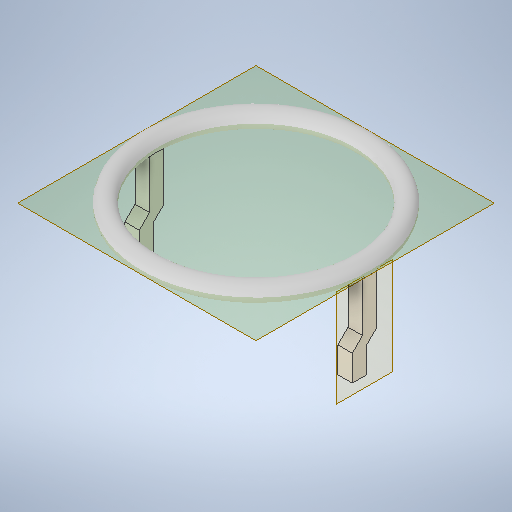
# Autodesk Inventor part: basket holder
Saved by Autodesk Inventor 2025.4 (Build 294407000, 407)
## iProperties
Created: 2026-03-21
Part Number: basket holder
Material: Generic
Document SubType Name: Modeling
Designer: Amir
Density: 1 g/cm^3
Appearance: Default
Author: Amir
Autodesk Inventor part; units mm, degrees
ref_plane "XZ Plane" through (0, 0, 0) normal (0, 1, 0) x (-1, 0, 0)
ref_plane "XY Plane" through (0, 0, 0) normal (0, 0, 1) x (1, 0, 0)
sketch "Sketch1" plane through (0, 0, 0) normal (0, 0, 1) x (1, 0, 0)
  circle A0 centre (0, 29.5) radius 2.5
  line L0 (-6.3664, 0) -> (5.4497, 0)
  point P0 (0, 0)
  dimension "d2" = 5
  dimension "d11" = 29.5
  constraints: 2 end point, 1 centre point, 1 horizontal
  measures "d2" diameter of A0
  measures "d11" distance from line of A0.centre L0
revolve "Revolution1" add sketch "Sketch1" angle 360 about axis through (-6.3664, 0, 0) along (1, 0, 0)
ref_plane "Work Plane1" through (0, 0, 0) normal (1, 0, 0) x (0, 1, 0)
sketch "Sketch2" plane through (0, 0, 0) normal (1, 0, 0) x (0, 1, 0)
  line L0 (2, -27.5) -> (-2, -27.5)
  line L1 (-2, -27.5) -> (-2, -31.5)
  line L2 (-2, -31.5) -> (2, -31.5)
  line L3 (2, -31.5) -> (2, -27.5)
  line L4 (2, -27.5) -> (-2, -31.5) construction
  line L5 (-2, -27.5) -> (2, -31.5) construction
  line L6 (2, 31.5) -> (-2, 31.5)
  line L7 (-2, 31.5) -> (-2, 27.5)
  line L8 (-2, 27.5) -> (2, 27.5)
  line L9 (2, 27.5) -> (2, 31.5)
  line L10 (2, 31.5) -> (-2, 27.5) construction
  line L11 (-2, 31.5) -> (2, 27.5) construction
  point P0 (0, 0)
  dimension "d13" = 4
  dimension "d14" = 4
  dimension "d15" = 4
  dimension "d16" = 4
  constraints: 24 end point, 4 parallel, 2 horizontal, 2 perpendicular
  measures "d13" distance of L2.end L1.end
  measures "d14" distance of L1.end L0.end
  measures "d15" distance of L8.end L7.end
  measures "d16" distance of L7.end L6.end
extrude "Extrusion2" add sketch "Sketch2" along normal blind 15
ref_plane "Work Plane3" through (15, 2, -31.5) normal (0, 0, -1) x (-1, 0, 0)
sketch "Sketch4" plane through (15, 2, -31.5) normal (0, 0, -1) x (-1, 0, 0)
  line L0 (0, -4) -> (0, 0) projected
  line L1 (0, 0) -> (-2.8284, 2.8284)
  line L2 (0, -4) -> (-2.8284, -1.1716)
  line L3 (-10, 6.652) -> (-10, -6.5658)
  line L4 (-2.8284, 2.8284) -> (-10, 2.8284)
  line L5 (-2.8284, -1.1716) -> (-10, -1.1716)
  line L6 (0, 0) -> (0, -4)
  point P0 (15, -2)
  dimension "d20" = 4
  dimension "d21" = 4
  dimension "d22" = 10
  dimension "d23" = 45
  constraints: 12 end point, 2 equal length, 2 perpendicular, 2 point on line, 1 vertical
  measures "d20" distance of L0.end L1.end
  measures "d21" distance of L0.start L2.end
  measures "d22" distance between parallel lines of L3 L0
  measures "d23" angle of L3 L1
extrude "Extrusion3" add sketch "Sketch4" against normal blind 63
extrude "Extrusion4" cut sketch "Sketch4" against normal blind 59
extrude "Extrusion5" add sketch "Sketch4" against normal blind 4
body "Solid1"
